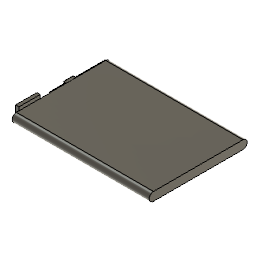
Battery (Autodesk Fusion 360 design; units mm, degrees)
Autodesk Fusion 360 part; units mm, degrees
sketch "Sketch1" plane through (0, 0, 0) normal (0, 0, 1) x (1, 0, 0)
  line L0 (0, 0) -> (79.58, 0)
  line L1 (79.58, 0) -> (79.58, 57)
  line L2 (79.58, 57) -> (0, 57)
  line L3 (0, 57) -> (0, 0)
  dimension "d1" = 79.58
  dimension "d2" = 57
  constraint horizontal L0
  constraint vertical L1
  constraint horizontal L2
  constraint vertical L3
  constraint coincident L0.start L3.end
  measures "d1" distance of L0.start L0.end
  measures "d2" distance of L0.start L2.end
extrude "Extrude1" add sketch "Sketch1" along normal blind 5
fillet "Fillet1" radius 2.5 4 edges at (39.79, 0, 5) (39.79, 0, 0) (39.79, 57, 5) (39.79, 57, 0)
sketch "Sketch2" plane through (0, 0, 0) normal (-1, 0, 0) x (0, -1, 0)
  arc A0 (-54.5, 5) -> (-54.5, 0) centre (-54.5, 2.5) ccw
  line L0 (-54.5, 0) -> (-2.5, 0)
  arc A1 (-2.5, 0) -> (-2.5, 5) centre (-2.5, 2.5) ccw
  line L1 (-2.5, 5) -> (-54.5, 5)
  line L2 (-54.5, 5) -> (-22, 5)
  line L3 (-22, 5) -> (-22, 0)
  line L4 (-22, 0) -> (-54.5, 0)
  arc A2 (-54.5, 5) -> (-54.5, 0) centre (-54.5, 2.5) ccw
  dimension "d7" = 5
  dimension "d8" = 32.5
  constraint concentric A0 A2
  constraint coincident A0.start L1.end
  constraint parallel L1 L2
  constraint coincident L0 L3.end
  constraint perpendicular L0 L3
  constraint coincident A0.end L0.start
  measures "d7" diameter of A2
  measures "d8" distance of A0.start L2.end
extrude "Extrude2" add sketch "Sketch2" along normal blind 0.3 contours A0 L0 L1 L2 L3 L4 A2
sketch "Sketch4" plane through (-0.3, 0, 0) normal (-1, 0, 0) x (0, -1, 0)
  line L0 (-22, 5) -> (-54.5, 5)
  arc A0 (-54.5, 5) -> (-54.5, 0) centre (-54.5, 2.5) ccw
  line L1 (-54.5, 0) -> (-22, 0)
  line L2 (-22, 0) -> (-22, 5)
  line L3 (-54.5, 0) -> (-22, 0)
  line L4 (-22, 0) -> (-22, 0.25)
  line L5 (-22, 0.25) -> (-54.5, 0.25)
  line L6 (-54.5, 0.25) -> (-54.5, 0)
  line L7 (-59.156, 2.5) -> (0.7958, 2.5) construction
  line L8 (-54.5, 5) -> (-22, 5)
  line L9 (-22, 5) -> (-22, 4.75)
  line L10 (-22, 4.75) -> (-54.5, 4.75)
  line L11 (-54.5, 4.75) -> (-54.5, 5)
  dimension "d11" = 0.25
  constraint horizontal L3
  constraint vertical L4
  constraint horizontal L5
  constraint vertical L6
  constraint coincident L2 L4.end
  constraint coincident A0.end L1.start
  constraint parallel L5 L7
  constraint symmetric A0.end L7 L0.end
  constraint symmetric L1.end L7 L0.start
  constraint symmetric L4.end L7 L9.end
  constraint symmetric L5.end L7 L10.end
  measures "d11" distance of A0.end L5.end
extrude "Extrude3" add sketch "Sketch4" along normal blind 0.35 contours L0 L2 L8 L9 L10 L11 | L1 L2 L3 L4 L5 L6
sketch "Sketch5" plane through (-0.65, 0, 0) normal (-1, 0, 0) x (0, -1, 0)
  line L0 (-54.5, 0) -> (-22, 0)
  line L1 (-22, 0) -> (-22, 0.25)
  line L2 (-31.55, 0.25) -> (-37.35, 0.25)
  line L3 (-37.35, 0.25) -> (-37.35, 0)
  line L4 (-37.35, 0) -> (-31.55, 0)
  line L5 (-31.55, 0) -> (-31.55, 0.25)
  line L6 (-54.5, 0.25) -> (-54.5, 0)
  line L7 (-22, 0.25) -> (-54.5, 0.25)
  line L8 (-58.264, 2.5) -> (4.0505, 2.5) construction
  line L9 (-22, 5) -> (-54.5, 5) construction
  line L10 (-31.55, 4.75) -> (-37.35, 4.75)
  line L11 (-37.35, 4.75) -> (-37.35, 5)
  line L12 (-37.35, 5) -> (-31.55, 5)
  line L13 (-31.55, 5) -> (-31.55, 4.75)
  dimension "d18" = 5.8
  dimension "d19" = 2.5
  dimension "d20" = 2.5
  constraint horizontal L2
  constraint vertical L3
  constraint horizontal L4
  constraint vertical L5
  constraint coincident L0 L3.end
  constraint parallel L0 L8
  constraint symmetric L2.start L8 L10.start
  constraint symmetric L2.end L8 L10.end
  constraint symmetric L3.end L8 L11.end
  constraint symmetric L4.end L8 L12.end
  measures "d18" distance of L2.start L2.end
  measures "d19" distance of L0 L8
  measures "d20" distance of L8 L9
extrude "Extrude4" add sketch "Sketch5" along normal blind 1.25 contours L0 L2 L3 L4 L5 L7 | L10 L11 L12 L13
sketch "Sketch6" plane through (0, 0, 0) normal (-1, 0, 0) x (0, -1, 0)
  line L0 (-22, 5) -> (-22, 0)
  line L1 (-22, 0) -> (-2.5, 0)
  arc A0 (-2.5, 0) -> (-2.5, 5) centre (-2.5, 2.5) ccw
  line L2 (-2.5, 5) -> (-22, 5)
  line L3 (-4, 7) -> (-16.4, 7)
  line L4 (-16.4, 7) -> (-16.4, 0)
  line L5 (-16.4, 0) -> (-4, 0)
  line L6 (-4, 0) -> (-4, 7)
  line L7 (0, 8.6382) -> (0, -2.5126) construction
  dimension "d21" = 4
  dimension "d22" = 12.4
  dimension "d23" = 2
  constraint horizontal L3
  constraint vertical L4
  constraint horizontal L5
  constraint vertical L6
  constraint coincident L1 L4.end
  constraint vertical L7
  constraint coincident origin L7
  measures "d21" distance of L6 L7
  measures "d22" distance of L3.start L3.end
  measures "d23" distance of L2 L3
extrude "Extrude5" add sketch "Sketch6" along normal blind 2 contours L2 L3 L4 L6 | L1 L2 L4 L5 L6
sketch "Sketch7" plane through (-0.3, 0, 0) normal (-1, 0, 0) x (0, -1, 0)
  line L0 (-22, 4.75) -> (-54.5, 4.75)
  line L1 (-54.5, 4.75) -> (-54.5, 5)
  arc A0 (-54.5, 5) -> (-54.5, 0) centre (-54.5, 2.5) ccw
  line L2 (-54.5, 0) -> (-54.5, 0.25)
  line L3 (-54.5, 0.25) -> (-22, 0.25)
  line L4 (-22, 0.25) -> (-22, 4.75)
  line L5 (-37.55, 4.25) -> (-31.55, 4.25)
  line L6 (-31.55, 4.25) -> (-31.55, 0.75)
  line L7 (-31.55, 0.75) -> (-37.55, 0.75)
  line L8 (-37.55, 0.75) -> (-37.55, 4.25)
  line L9 (-59.3246, 2.5) -> (-29.1063, 2.5) construction
  line L10 (-31.55, 7.2978) -> (-31.55, -1.062) construction
  point P0 (-31.55, 5)
  dimension "d26" = 6
  dimension "d27" = 3.5
  dimension "d28" = 1.75
  constraint horizontal L5
  constraint vertical L6
  constraint horizontal L7
  constraint vertical L8
  constraint horizontal L9
  constraint coincident A0.centre L9
  constraint perpendicular L0 L10
  constraint coincident L10 P0
  constraint collinear L6 L10
  measures "d26" distance of L5.start L5.end
  measures "d27" distance of L5.start L7.end
  measures "d28" distance of L5 L9
extrude "Extrude7" add sketch "Sketch7" along normal blind 1.4 contours L5 L6 L7 L8
sketch "Sketch8" plane through (-0.3, 0, 0) normal (-1, 0, 0) x (0, -1, 0)
  line L0 (-22, 4.75) -> (-54.5, 4.75)
  line L1 (-54.5, 4.75) -> (-54.5, 5)
  arc A0 (-54.5, 5) -> (-54.5, 0) centre (-54.5, 2.5) ccw
  line L2 (-54.5, 0) -> (-54.5, 0.25)
  line L3 (-54.5, 0.25) -> (-22, 0.25)
  line L4 (-22, 0.25) -> (-22, 4.75)
  line L5 (-25.4, 4) -> (-43.1, 4)
  line L6 (-43.1, 4) -> (-43.1, 1)
  line L7 (-43.1, 1) -> (-25.4, 1)
  line L8 (-25.4, 1) -> (-25.4, 4)
  line L9 (-57, 2.5) -> (-22, 2.5) construction
  line L10 (-37.55, 0.75) -> (-37.55, 4.25)
  line L11 (-37.55, 4.25) -> (-31.55, 4.25)
  line L12 (-31.55, 4.25) -> (-31.55, 0.75)
  line L13 (-31.55, 0.75) -> (-37.55, 0.75)
  dimension "d29" = 1.5
  dimension "d30" = 3
  dimension "d31" = 17.7
  dimension "d32" = 3.4
  constraint horizontal L5
  constraint vertical L6
  constraint horizontal L7
  constraint vertical L8
  constraint midpoint L4 L9.end
  constraint perpendicular L4 L9
  constraint midpoint A0 L9.start
  measures "d29" distance of L5 L9
  measures "d30" distance of L5.end L6.end
  measures "d31" distance of L5.start L5.end
  measures "d32" distance of L4 L8
extrude "Extrude6" add sketch "Sketch8" along normal blind 0.65 contours L5 L7 L8 L12 | L5 L7 L10 L12 | L5 L6 L7 L10
equation "d8 = 35 mm - ( d7 / 2 )"
equation "d28 = d27 / 2"
equation "d29 = d30 / 2"
